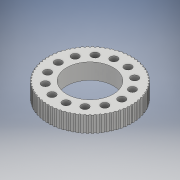
# Autodesk Inventor part: poulie 72 dents
Saved by Autodesk Inventor 2018.1 (Build 221171000, 171)
## iProperties
Created: 2022-05-13
Part Number: poulie 72 dents
Material: Generic
Document SubType Name: Modeling
Designer: Bureau
Density: 1 g/cm^3
Appearance: Default
Author: Bureau
Autodesk Inventor part; units mm, degrees
ref_plane "YZ Plane" through (0, 0, 0) normal (1, 0, 0) x (0, 1, 0)
ref_plane "XZ Plane" through (0, 0, 0) normal (0, 1, 0) x (-1, 0, 0)
ref_plane "XY Plane" through (0, 0, 0) normal (0, 0, 1) x (1, 0, 0)
sketch "Sketch1" plane through (0, 0, 0) normal (0, 0, 1) x (1, 0, 0)
  circle A0 centre (0, 0) radius 19
  arc A1 (-0.75, 34.3668) -> (0.75, 34.3668) centre (0, 34.375) ccw
  arc A2 (-3.7424, 34.1707) -> (-2.2482, 34.3014) centre (-2.996, 34.2442) ccw
  arc A3 (-6.7063, 33.7145) -> (-5.2292, 33.9749) centre (-5.9692, 33.8528) ccw
  arc A4 (-9.6192, 33.0017) -> (-8.1704, 33.3899) centre (-8.8969, 33.2037) ccw
  arc A5 (-12.4589, 32.0377) -> (-11.0494, 32.5507) centre (-11.7569, 32.3019) ccw
  arc A6 (-15.2037, 30.83) -> (-13.8444, 31.4639) centre (-14.5275, 31.1543) ccw
  arc A7 (-17.8329, 29.3876) -> (-16.5339, 30.1375) centre (-17.1875, 29.7696) ccw
  arc A8 (-20.3263, 27.7215) -> (-19.0977, 28.5818) centre (-19.7167, 28.1584) ccw
  arc A9 (-22.6651, 25.8444) -> (-21.5161, 26.8086) centre (-22.0958, 26.3328) ccw
  arc A10 (-24.8313, 23.7707) -> (-23.7707, 24.8313) centre (-24.3068, 24.3068) ccw
  arc A11 (-26.8086, 21.5161) -> (-25.8444, 22.6651) centre (-26.3328, 22.0958) ccw
  arc A12 (-28.5818, 19.0977) -> (-27.7215, 20.3263) centre (-28.1584, 19.7167) ccw
  arc A13 (-30.1375, 16.5339) -> (-29.3876, 17.8329) centre (-29.7696, 17.1875) ccw
  arc A14 (-31.4639, 13.8444) -> (-30.83, 15.2037) centre (-31.1543, 14.5275) ccw
  arc A15 (-32.5507, 11.0494) -> (-32.0377, 12.4589) centre (-32.3019, 11.7569) ccw
  arc A16 (-33.3899, 8.1704) -> (-33.0017, 9.6192) centre (-33.2037, 8.8969) ccw
  arc A17 (-33.9749, 5.2292) -> (-33.7145, 6.7063) centre (-33.8528, 5.9692) ccw
  arc A18 (-34.3014, 2.2482) -> (-34.1707, 3.7424) centre (-34.2442, 2.996) ccw
  arc A19 (-34.3668, -0.75) -> (-34.3668, 0.75) centre (-34.375, 0) ccw
  arc A20 (-34.1707, -3.7424) -> (-34.3014, -2.2482) centre (-34.2442, -2.996) ccw
  arc A21 (-33.7145, -6.7063) -> (-33.9749, -5.2292) centre (-33.8528, -5.9692) ccw
  arc A22 (-33.0017, -9.6192) -> (-33.3899, -8.1704) centre (-33.2037, -8.8969) ccw
  arc A23 (-32.0377, -12.4589) -> (-32.5507, -11.0494) centre (-32.3019, -11.7569) ccw
  arc A24 (-30.83, -15.2037) -> (-31.4639, -13.8444) centre (-31.1543, -14.5275) ccw
  arc A25 (-29.3876, -17.8329) -> (-30.1375, -16.5339) centre (-29.7696, -17.1875) ccw
  arc A26 (-27.7215, -20.3263) -> (-28.5818, -19.0977) centre (-28.1584, -19.7167) ccw
  arc A27 (-25.8444, -22.6651) -> (-26.8086, -21.5161) centre (-26.3328, -22.0958) ccw
  arc A28 (-23.7707, -24.8313) -> (-24.8313, -23.7707) centre (-24.3068, -24.3068) ccw
  arc A29 (-21.5161, -26.8086) -> (-22.6651, -25.8444) centre (-22.0958, -26.3328) ccw
  arc A30 (-19.0977, -28.5818) -> (-20.3263, -27.7215) centre (-19.7167, -28.1584) ccw
  arc A31 (-16.5339, -30.1375) -> (-17.8329, -29.3876) centre (-17.1875, -29.7696) ccw
  arc A32 (-13.8444, -31.4639) -> (-15.2037, -30.83) centre (-14.5275, -31.1543) ccw
  arc A33 (-11.0494, -32.5507) -> (-12.4589, -32.0377) centre (-11.7569, -32.3019) ccw
  arc A34 (-8.1704, -33.3899) -> (-9.6192, -33.0017) centre (-8.8969, -33.2037) ccw
  arc A35 (-5.2292, -33.9749) -> (-6.7063, -33.7145) centre (-5.9692, -33.8528) ccw
  arc A36 (-2.2482, -34.3014) -> (-3.7424, -34.1707) centre (-2.996, -34.2442) ccw
  arc A37 (0.75, -34.3668) -> (-0.75, -34.3668) centre (0, -34.375) ccw
  arc A38 (3.7424, -34.1707) -> (2.2482, -34.3014) centre (2.996, -34.2442) ccw
  arc A39 (6.7063, -33.7145) -> (5.2292, -33.9749) centre (5.9692, -33.8528) ccw
  arc A40 (9.6192, -33.0017) -> (8.1704, -33.3899) centre (8.8969, -33.2037) ccw
  arc A41 (12.4589, -32.0377) -> (11.0494, -32.5507) centre (11.7569, -32.3019) ccw
  arc A42 (15.2037, -30.83) -> (13.8444, -31.4639) centre (14.5275, -31.1543) ccw
  arc A43 (17.8329, -29.3876) -> (16.5339, -30.1375) centre (17.1875, -29.7696) ccw
  arc A44 (20.3263, -27.7215) -> (19.0977, -28.5818) centre (19.7167, -28.1584) ccw
  arc A45 (22.6651, -25.8444) -> (21.5161, -26.8086) centre (22.0958, -26.3328) ccw
  arc A46 (24.8313, -23.7707) -> (23.7707, -24.8313) centre (24.3068, -24.3068) ccw
  arc A47 (26.8086, -21.5161) -> (25.8444, -22.6651) centre (26.3328, -22.0958) ccw
  arc A48 (28.5818, -19.0977) -> (27.7215, -20.3263) centre (28.1584, -19.7167) ccw
  arc A49 (30.1375, -16.5339) -> (29.3876, -17.8329) centre (29.7696, -17.1875) ccw
  arc A50 (31.4639, -13.8444) -> (30.83, -15.2037) centre (31.1543, -14.5275) ccw
  arc A51 (32.5507, -11.0494) -> (32.0377, -12.4589) centre (32.3019, -11.7569) ccw
  arc A52 (33.3899, -8.1704) -> (33.0017, -9.6192) centre (33.2037, -8.8969) ccw
  arc A53 (33.9749, -5.2292) -> (33.7145, -6.7063) centre (33.8528, -5.9692) ccw
  arc A54 (34.3014, -2.2482) -> (34.1707, -3.7424) centre (34.2442, -2.996) ccw
  arc A55 (34.3668, 0.75) -> (34.3668, -0.75) centre (34.375, 0) ccw
  arc A56 (34.1707, 3.7424) -> (34.3014, 2.2482) centre (34.2442, 2.996) ccw
  arc A57 (33.7145, 6.7063) -> (33.9749, 5.2292) centre (33.8528, 5.9692) ccw
  arc A58 (33.0017, 9.6192) -> (33.3899, 8.1704) centre (33.2037, 8.8969) ccw
  arc A59 (32.0377, 12.4589) -> (32.5507, 11.0494) centre (32.3019, 11.7569) ccw
  arc A60 (30.83, 15.2037) -> (31.4639, 13.8444) centre (31.1543, 14.5275) ccw
  arc A61 (29.3876, 17.8329) -> (30.1375, 16.5339) centre (29.7696, 17.1875) ccw
  arc A62 (27.7215, 20.3263) -> (28.5818, 19.0977) centre (28.1584, 19.7167) ccw
  arc A63 (25.8444, 22.6651) -> (26.8086, 21.5161) centre (26.3328, 22.0958) ccw
  arc A64 (23.7707, 24.8313) -> (24.8313, 23.7707) centre (24.3068, 24.3068) ccw
  arc A65 (21.5161, 26.8086) -> (22.6651, 25.8444) centre (22.0958, 26.3328) ccw
  arc A66 (19.0977, 28.5818) -> (20.3263, 27.7215) centre (19.7167, 28.1584) ccw
  arc A67 (16.5339, 30.1375) -> (17.8329, 29.3876) centre (17.1875, 29.7696) ccw
  arc A68 (13.8444, 31.4639) -> (15.2037, 30.83) centre (14.5275, 31.1543) ccw
  arc A69 (11.0494, 32.5507) -> (12.4589, 32.0377) centre (11.7569, 32.3019) ccw
  arc A70 (8.1704, 33.3899) -> (9.6192, 33.0017) centre (8.8969, 33.2037) ccw
  arc A71 (5.2292, 33.9749) -> (6.7063, 33.7145) centre (5.9692, 33.8528) ccw
  arc A72 (2.2482, 34.3014) -> (3.7424, 34.1707) centre (2.996, 34.2442) ccw
  arc A73 (2.2482, 34.3014) -> (0.75, 34.3668) centre (0, 0) ccw
  arc A74 (5.2292, 33.9749) -> (3.7424, 34.1707) centre (0, 0) ccw
  arc A75 (8.1704, 33.3899) -> (6.7063, 33.7145) centre (0, 0) ccw
  arc A76 (13.8444, 31.4639) -> (12.4589, 32.0377) centre (0, 0) ccw
  arc A77 (11.0494, 32.5507) -> (9.6192, 33.0017) centre (0, 0) ccw
  arc A78 (16.5339, 30.1375) -> (15.2037, 30.83) centre (0, 0) ccw
  arc A79 (19.0977, 28.5818) -> (17.8329, 29.3876) centre (0, 0) ccw
  arc A80 (21.5161, 26.8086) -> (20.3263, 27.7215) centre (0, 0) ccw
  arc A81 (23.7707, 24.8313) -> (22.6651, 25.8444) centre (0, 0) ccw
  arc A82 (25.8444, 22.6651) -> (24.8313, 23.7707) centre (0, 0) ccw
  arc A83 (27.7215, 20.3263) -> (26.8086, 21.5161) centre (0, 0) ccw
  arc A84 (29.3876, 17.8329) -> (28.5818, 19.0977) centre (0, 0) ccw
  arc A85 (30.83, 15.2037) -> (30.1375, 16.5339) centre (0, 0) ccw
  arc A86 (32.0377, 12.4589) -> (31.4639, 13.8444) centre (0, 0) ccw
  arc A87 (33.0017, 9.6192) -> (32.5507, 11.0494) centre (0, 0) ccw
  arc A88 (33.7145, 6.7063) -> (33.3899, 8.1704) centre (0, 0) ccw
  arc A89 (34.1707, 3.7424) -> (33.9749, 5.2292) centre (0, 0) ccw
  arc A90 (34.3668, 0.75) -> (34.3014, 2.2482) centre (0, 0) ccw
  arc A91 (34.3014, -2.2482) -> (34.3668, -0.75) centre (0, 0) ccw
  arc A92 (33.9749, -5.2292) -> (34.1707, -3.7424) centre (0, 0) ccw
  arc A93 (33.3899, -8.1704) -> (33.7145, -6.7063) centre (0, 0) ccw
  arc A94 (32.5507, -11.0494) -> (33.0017, -9.6192) centre (0, 0) ccw
  arc A95 (31.4639, -13.8444) -> (32.0377, -12.4589) centre (0, 0) ccw
  arc A96 (30.1375, -16.5339) -> (30.83, -15.2037) centre (0, 0) ccw
  arc A97 (28.5818, -19.0977) -> (29.3876, -17.8329) centre (0, 0) ccw
  arc A98 (26.8086, -21.5161) -> (27.7215, -20.3263) centre (0, 0) ccw
  arc A99 (24.8313, -23.7707) -> (25.8444, -22.6651) centre (0, 0) ccw
  arc A100 (22.6651, -25.8444) -> (23.7707, -24.8313) centre (0, 0) ccw
  arc A101 (20.3263, -27.7215) -> (21.5161, -26.8086) centre (0, 0) ccw
  arc A102 (17.8329, -29.3876) -> (19.0977, -28.5818) centre (0, 0) ccw
  arc A103 (15.2037, -30.83) -> (16.5339, -30.1375) centre (0, 0) ccw
  arc A104 (12.4589, -32.0377) -> (13.8444, -31.4639) centre (0, 0) ccw
  arc A105 (9.6192, -33.0017) -> (11.0494, -32.5507) centre (0, 0) ccw
  arc A106 (6.7063, -33.7145) -> (8.1704, -33.3899) centre (0, 0) ccw
  arc A107 (3.7424, -34.1707) -> (5.2292, -33.9749) centre (0, 0) ccw
  arc A108 (0.75, -34.3668) -> (2.2482, -34.3014) centre (0, 0) ccw
  arc A109 (-2.2482, -34.3014) -> (-0.75, -34.3668) centre (0, 0) ccw
  arc A110 (-5.2292, -33.9749) -> (-3.7424, -34.1707) centre (0, 0) ccw
  arc A111 (-8.1704, -33.3899) -> (-6.7063, -33.7145) centre (0, 0) ccw
  arc A112 (-11.0494, -32.5507) -> (-9.6192, -33.0017) centre (0, 0) ccw
  arc A113 (-13.8444, -31.4639) -> (-12.4589, -32.0377) centre (0, 0) ccw
  arc A114 (-16.5339, -30.1375) -> (-15.2037, -30.83) centre (0, 0) ccw
  arc A115 (-19.0977, -28.5818) -> (-17.8329, -29.3876) centre (0, 0) ccw
  arc A116 (-21.5161, -26.8086) -> (-20.3263, -27.7215) centre (0, 0) ccw
  arc A117 (-23.7707, -24.8313) -> (-22.6651, -25.8444) centre (0, 0) ccw
  arc A118 (-25.8444, -22.6651) -> (-24.8313, -23.7707) centre (0, 0) ccw
  arc A119 (-27.7215, -20.3263) -> (-26.8086, -21.5161) centre (0, 0) ccw
  arc A120 (-29.3876, -17.8329) -> (-28.5818, -19.0977) centre (0, 0) ccw
  arc A121 (-30.83, -15.2037) -> (-30.1375, -16.5339) centre (0, 0) ccw
  arc A122 (-32.0377, -12.4589) -> (-31.4639, -13.8444) centre (0, 0) ccw
  arc A123 (-33.0017, -9.6192) -> (-32.5507, -11.0494) centre (0, 0) ccw
  arc A124 (-33.7145, -6.7063) -> (-33.3899, -8.1704) centre (0, 0) ccw
  arc A125 (-34.1707, -3.7424) -> (-33.9749, -5.2292) centre (0, 0) ccw
  arc A126 (-33.9749, 5.2292) -> (-34.1707, 3.7424) centre (0, 0) ccw
  arc A127 (-33.3899, 8.1704) -> (-33.7145, 6.7063) centre (0, 0) ccw
  arc A128 (-32.5507, 11.0494) -> (-33.0017, 9.6192) centre (0, 0) ccw
  arc A129 (-31.4639, 13.8444) -> (-32.0377, 12.4589) centre (0, 0) ccw
  arc A130 (-30.1375, 16.5339) -> (-30.83, 15.2037) centre (0, 0) ccw
  arc A131 (-28.5818, 19.0977) -> (-29.3876, 17.8329) centre (0, 0) ccw
  arc A132 (-26.8086, 21.5161) -> (-27.7215, 20.3263) centre (0, 0) ccw
  arc A133 (-24.8313, 23.7707) -> (-25.8444, 22.6651) centre (0, 0) ccw
  arc A134 (-22.6651, 25.8444) -> (-23.7707, 24.8313) centre (0, 0) ccw
  arc A135 (-20.3263, 27.7215) -> (-21.5161, 26.8086) centre (0, 0) ccw
  arc A136 (-17.8329, 29.3876) -> (-19.0977, 28.5818) centre (0, 0) ccw
  arc A137 (-15.2037, 30.83) -> (-16.5339, 30.1375) centre (0, 0) ccw
  arc A138 (-12.4589, 32.0377) -> (-13.8444, 31.4639) centre (0, 0) ccw
  arc A139 (-9.6192, 33.0017) -> (-11.0494, 32.5507) centre (0, 0) ccw
  arc A140 (-6.7063, 33.7145) -> (-8.1704, 33.3899) centre (0, 0) ccw
  arc A141 (-0.75, 34.3668) -> (-2.2482, 34.3014) centre (0, 0) ccw
  arc A142 (-3.7424, 34.1707) -> (-5.2292, 33.9749) centre (0, 0) ccw
  arc A143 (-34.3014, 2.2482) -> (-34.3668, 0.75) centre (0, 0) ccw
  arc A144 (-34.3668, -0.75) -> (-34.3014, -2.2482) centre (0, 0) ccw
  line L0 (0, 0) -> (26, 0)
  circle A145 centre (26, 0) radius 3
  circle A146 centre (23.4252, 11.281) radius 3
  circle A147 centre (16.2107, 20.3276) radius 3
  circle A148 centre (5.7855, 25.3481) radius 3
  circle A149 centre (-5.7855, 25.3481) radius 3
  circle A150 centre (-16.2107, 20.3276) radius 3
  circle A151 centre (-23.4252, 11.281) radius 3
  circle A152 centre (-26, 0) radius 3
  circle A153 centre (-23.4252, -11.281) radius 3
  circle A154 centre (-16.2107, -20.3276) radius 3
  circle A155 centre (-5.7855, -25.3481) radius 3
  circle A156 centre (5.7855, -25.3481) radius 3
  circle A157 centre (16.2107, -20.3276) radius 3
  circle A158 centre (23.4252, -11.281) radius 3
  dimension "d0" = 38
  dimension "d2" = 1.5
  dimension "d5" = 360
  dimension "d9" = 26
  dimension "d10" = 6
  dimension "d13" = 360
  constraints: 144 point on circle, 87 centre point, 3 horizontal, 2 coincident, 1 end point, 535 other
  measures "d0" diameter of A0
  measures "d2" diameter of A1
  measures "d10" diameter of A145
extrude "Extrusion2" add sketch "Sketch1" along normal blind 13
body "Solid2"
